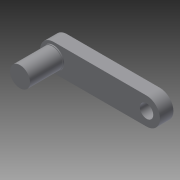
# Autodesk Inventor part: Frame
Saved by Autodesk Inventor 2018 (Build 220112000, 112)
## iProperties
Created: 2018-01-20
Part Number: Frame
Material: Generic
Document SubType Name: Modeling
Designer: Rus
Density: 1 g/cm^3
Appearance: Default
Author: Rus
Autodesk Inventor part; units mm, degrees
ref_plane "YZ Plane" through (0, 0, 0) normal (1, 0, 0) x (0, 1, 0)
ref_plane "XZ Plane" through (0, 0, 0) normal (0, 1, 0) x (-1, 0, 0)
ref_plane "XY Plane" through (0, 0, 0) normal (0, 0, 1) x (1, 0, 0)
sketch "Sketch1" plane through (0, 0, 0) normal (0, 0, 1) x (1, 0, 0)
  circle A0 centre (-43.9941, 0) radius 9.525
  circle A1 centre (43.9941, 0) radius 6.35
  line L0 (43.9941, 0) -> (-43.9941, 0) construction
  line L1 (43.9941, 12.7) -> (-43.9941, 12.7)
  line L2 (-43.9941, -12.7) -> (43.9941, -12.7)
  arc A2 (43.9941, -12.7) -> (43.9941, 12.7) centre (43.9941, 0) ccw
  arc A3 (-43.9941, 12.7) -> (-43.9941, -12.7) centre (-43.9941, 0) ccw
  point P0 (0, 0)
  point P1 (0, 0)
  dimension "d10" = 12.7
  dimension "d11" = 19.05
  dimension "d12" = 87.9881
  dimension "d13" = 12.7
  constraints: 8 end point, 4 centre point, 4 point on circle, 4 tangent, 1 coincident, 1 horizontal, 1 midpoint, 1 parallel
  measures "d10" diameter of A1
  measures "d11" diameter of A0
  measures "d12" distance of L0.start L0.end
  measures "d13" distance of L2.start L0.end
extrude "Extrusion1" add sketch "Sketch1" against normal blind 12.7
extrude "Extrusion2" add sketch "Sketch1" along normal blind 31.6653 and the other way blind 12.7 contours A0
sketch "Sketch2" plane through (0, 0, 0) normal (0, 0, 1) x (1, 0, 0)
  circle A0 centre (-43.9941, 0) radius 9.525 projected
  circle A1 centre (-43.9941, 0) radius 10.033
  point P0 (0, 0)
  dimension "d20" = 20.066
  constraints: 1 centre point, 1 coincident
  measures "d20" diameter of A1
extrude "Extrusion3" add sketch "Sketch2" along normal blind 1
body "Solid1"
